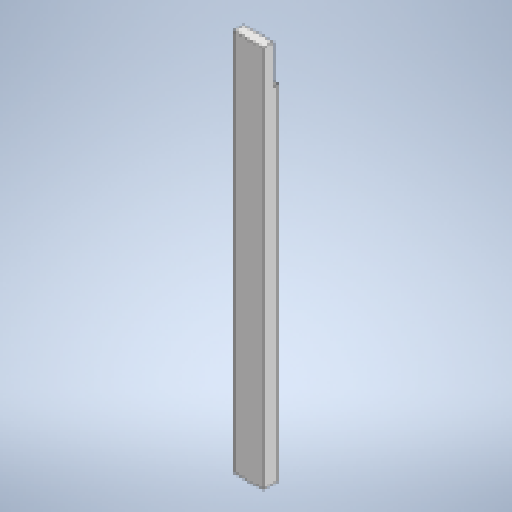
# Autodesk Inventor part: Нога для постели №2
Saved by Autodesk Inventor 2025 (Build 290162010, 162A)
## iProperties
Created: 2025-08-21
Part Number: Нога для постели №2
Material: Generic
Document SubType Name: Modeling
Designer: pokla
Density: 1 g/cm^3
Appearance: Default
Author: pokla
Autodesk Inventor part; units mm, degrees
ref_plane "YZ Plane" through (0, 0, 0) normal (1, 0, 0) x (0, 1, 0)
ref_plane "XZ Plane" through (0, 0, 0) normal (0, 1, 0) x (-1, 0, 0)
ref_plane "XY Plane" through (0, 0, 0) normal (0, 0, 1) x (1, 0, 0)
sketch "Sketch1" plane through (0, 0, 0) normal (0, 0, 1) x (1, 0, 0)
  line L0 (-30, 15) -> (30, 15)
  line L1 (30, 15) -> (30, -15)
  line L2 (30, -15) -> (-30, -15)
  line L3 (-30, -15) -> (-30, 15)
  line L4 (-30, 15) -> (30, -15) construction
  point P0 (0, 0)
  point P1 (0, 0)
  dimension "d0" = 60
  dimension "d1" = 30
  constraints: 10 end point, 2 parallel, 1 coincident, 1 horizontal, 1 midpoint, 1 perpendicular
  measures "d0" distance of L1.end L2.end
  measures "d1" distance of L2.end L0.start
extrude "Extrusion1" add sketch "Sketch1" along normal blind 779
sketch "Sketch2" plane through (30, -15, 0) normal (1, 0, 0) x (0, 0, -1)
  line L0 (0, 30) -> (-779, 30) projected
  line L1 (-779, 0) -> (-779, 30) projected
  line L2 (-779, 30) -> (-700, 30)
  line L3 (-700, 30) -> (-700, 20)
  line L4 (-700, 20) -> (-779, 20)
  line L5 (-779, 20) -> (-779, 30)
  point P0 (0, 15)
  dimension "d4" = 10
  dimension "d5" = 79
  constraints: 8 end point, 2 parallel, 1 horizontal, 1 perpendicular
  measures "d4" distance between parallel lines of L0 L4
  measures "d5" distance of L3.end L4.end
extrude "Extrusion2" cut sketch "Sketch2" against normal through all
body "Solid1"
